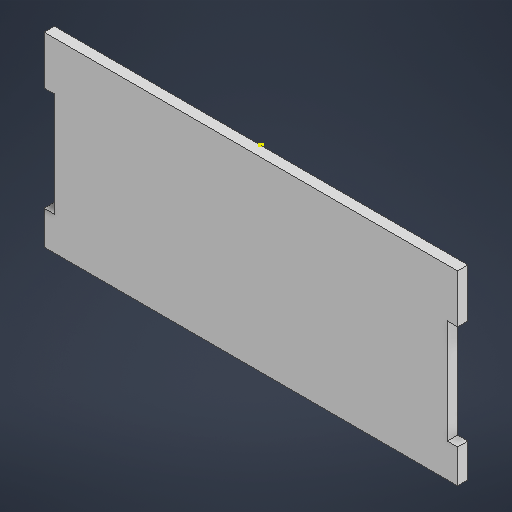
# Autodesk Inventor part: top inclinado
Saved by Autodesk Inventor 2026 (Build 300175050, 175E)
## iProperties
Created: 2025-08-08
Part Number: top inclinado
Material: Genérico
Document SubType Name: Modeling
Designer: EspacoMaker
Density: 1 g/cm^3
Appearance: Padrão
Author: EspacoMaker
Autodesk Inventor part; units mm, degrees
ref_plane "YZ Plane" through (0, 0, 0) normal (1, 0, 0) x (0, 1, 0)
ref_plane "XZ Plane" through (0, 0, 0) normal (0, 1, 0) x (-1, 0, 0)
ref_plane "XY Plane" through (0, 0, 0) normal (0, 0, 1) x (1, 0, 0)
sketch "Esboço1" plane through (0, 0, 0) normal (0, 0, 1) x (1, 0, 0)
  line L0 (60, -27) -> (-60, -27)
  line L1 (-60, -27) -> (-60, 27)
  line L2 (-60, 27) -> (60, 27)
  line L3 (60, 27) -> (60, -27)
  line L4 (60, -27) -> (-60, 27) construction
  line L5 (-60, -27) -> (60, 27) construction
  point P0 (0, 0)
  dimension "d0" = 120
  dimension "d1" = 54
  constraints: 12 end point, 2 midpoint, 2 parallel, 1 horizontal, 1 perpendicular
  measures "d0" distance of L1.end L2.end
  measures "d1" distance of L0.end L1.end
extrude "Extrusão1" add sketch "Esboço1" along normal blind 3
sketch "Esboço2" plane through (60, -27, 0) normal (1, 0, 0) x (0, 0, -1)
  line L0 (0, 54) -> (0, 43.9)
  line L1 (0, 54) -> (0, 0) projected
  line L2 (0, 0) -> (0, 9.75)
  line L3 (0, 9.75) -> (-3, 9.75)
  line L4 (-3, 9.75) -> (-3, 39.95)
  line L5 (-3, 39.95) -> (0, 39.95)
  line L6 (0, 39.95) -> (0, 9.75)
  point P0 (0, 27)
  point P1 (0, 39.95)
  point P2 (-1.5, 9.75)
  point P3 (-1.5, 39.95)
  dimension "d5" = 9.75
  dimension "d6" = 3
  dimension "d22" = 30.2
  constraints: 12 end point, 2 midpoint, 2 parallel, 2 point on line, 1 horizontal, 1 perpendicular
  measures "d5" distance of L1.end L2.end
  measures "d6" distance of L4.end L5.end
  measures "d22" distance of point (-1.5, 9.75) point (-1.5, 39.95)
extrude "Extrusão2" cut sketch "Esboço2" against normal blind 3
sketch "Esboço3" plane through (-60, -27, 0) normal (-1, 0, 0) x (0, 0, 1)
  line L0 (3, 39.95) -> (3, 54) projected
  line L1 (3, 54) -> (3, 39.95)
  line L2 (3, 0) -> (3, 9.75) projected
  line L3 (3, 0) -> (3, 9.75)
  line L4 (0, 39.95) -> (0, 9.75) projected
  line L5 (3, 9.75) -> (0, 9.75)
  line L6 (0, 9.75) -> (0, 39.95)
  line L7 (0, 39.95) -> (3, 39.95)
  line L8 (3, 39.95) -> (3, 9.75)
  point P0 (0, 27)
  constraints: 12 end point, 4 equal length, 1 horizontal, 1 perpendicular
extrude "Extrusão3" cut sketch "Esboço3" against normal blind 3
sketch "Esboço4" plane through (-60, 27, 0) normal (0, 1, 0) x (1, 0, 0)
  point P0 (60, 0)
